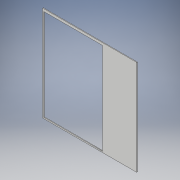
# Autodesk Inventor part: face-avant
Saved by Autodesk Inventor 2019 (Build 230136000, 136)
## iProperties
Created: 2018-12-30
Part Number: face-avant
Material: Générique
Document SubType Name: Modeling
Designer: pouey
Density: 1 g/cm^3
Appearance: Par défaut
Author: pouey
Autodesk Inventor part; units mm, degrees
ref_plane "YZ Plane" through (0, 0, 0) normal (1, 0, 0) x (0, 1, 0)
ref_plane "XZ Plane" through (0, 0, 0) normal (0, 1, 0) x (-1, 0, 0)
ref_plane "XY Plane" through (0, 0, 0) normal (0, 0, 1) x (1, 0, 0)
sketch "Esquisse1" plane through (0, 0, 0) normal (0, 0, 1) x (1, 0, 0)
  line L0 (0, 0) -> (400, 0)
  line L1 (400, 0) -> (400, 405)
  line L2 (400, 405) -> (0, 405)
  line L3 (0, 405) -> (0, 0)
  dimension "d0" = 400
  dimension "d1" = 405
  constraints: 8 end point, 2 parallel, 1 horizontal, 1 perpendicular
  measures "d0" distance of L1.end L2.end
  measures "d1" distance of L0.end L1.end
extrude "Extrusion1" add sketch "Esquisse1" along normal blind 3
sketch "Esquisse2" plane through (0, 0, 3) normal (0, 0, 1) x (1, 0, 0)
  line L0 (5, 395) -> (255, 395)
  line L1 (255, 395) -> (255, 5)
  line L2 (255, 5) -> (5, 5)
  line L3 (5, 5) -> (5, 395)
  line L4 (0, 0) -> (400, 0) projected
  line L5 (0, 405) -> (0, 0) projected
  dimension "d4" = 390
  dimension "d5" = 5
  dimension "d6" = 5
  dimension "d7" = 250
  constraints: 8 end point, 2 parallel, 1 horizontal, 1 perpendicular
  measures "d4" distance of L0.end L1.end
  measures "d5" distance between parallel lines of L4 L2
  measures "d6" distance between parallel lines of L5 L3
  measures "d7" distance between parallel lines of L3 L1
extrude "Extrusion2" cut sketch "Esquisse2" against normal blind 3
